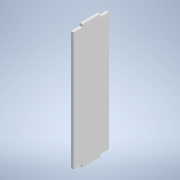
# Autodesk Inventor part: ACHTERRUIT
Saved by Autodesk Inventor 2021 (Build 250183000, 183)
## iProperties
Created: 2022-02-02
Part Number: ACHTERRUIT
Material: Generic
Document SubType Name: Modeling
Designer: ryan
Density: 1 g/cm^3
Appearance: Default
Author: ryan
Autodesk Inventor part; units mm, degrees
ref_plane "YZ Plane" through (0, 0, 0) normal (1, 0, 0) x (0, 1, 0)
ref_plane "XZ Plane" through (0, 0, 0) normal (0, 1, 0) x (-1, 0, 0)
ref_plane "XY Plane" through (0, 0, 0) normal (0, 0, 1) x (1, 0, 0)
sketch "Sketch1" plane through (0, 0, 0) normal (1, 0, 0) x (0, 1, 0)
  line L0 (0, 0) -> (-3, 0)
  line L1 (-3, 0) -> (67, 0)
  line L2 (67, 0) -> (67, -40)
  line L3 (67, -40) -> (-3, -40)
  line L4 (-3, -40) -> (-3, 0)
  line L5 (0, 0) -> (0, -10)
  line L6 (0, -10) -> (0, -30)
  line L7 (0, -30) -> (0, -40)
  line L8 (0, -30) -> (-3, -30)
  line L9 (0, -10) -> (-3, -10)
  dimension "d0" = 3
  dimension "d1" = 70
  dimension "d2" = 40
  dimension "d3" = 10
  dimension "d4" = 20
  constraints: 20 end point, 5 point on line, 3 perpendicular, 2 horizontal, 2 parallel, 1 vertical
  measures "d0" distance of L0.start L0.end
  measures "d1" distance of L2.end L3.end
  measures "d2" distance of L1.end L2.end
  measures "d3" distance of L0.start L5.end
  measures "d4" distance of L5.end L6.end
extrude "Extrusion1" add sketch "Sketch1" along normal blind 3 contours L1 L2 L3 L7 L6 L5 | L6 L8 L4 L9
mirror "Mirror1" about plane through (0, 67, -40) normal (0, 1, 0) of "Extrusion1"
body "Solid1"
